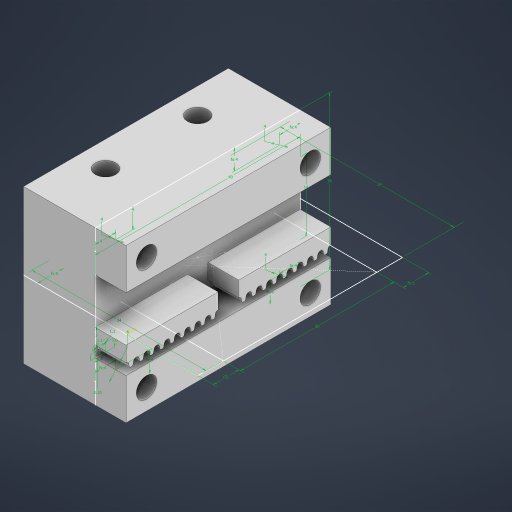
# Autodesk Inventor part: LRT_Back
Saved by Autodesk Inventor 2024.2 (Build 282272000, 272)
## iProperties
Created: 2024-09-29
Part Number: LRT_Back
Material: Generic
Document SubType Name: Modeling
Designer: jerem
Density: 1 g/cm^3
Appearance: Default
Author: jerem
## iProperties of the stored document linearRailToolhead_3DPrint.ipt
Created: 2024-09-29
Part Number: linearRailToolhead_3DPrint
Material: Generic
Document SubType Name: Modeling
Designer: jerem
Density: 1 g/cm^3
Appearance: Default
Author: jerem
Autodesk Inventor part; units mm, degrees
ref_plane "YZ Plane" through (0, 0, 0) normal (1, 0, 0) x (0, 1, 0)
ref_plane "XZ Plane" through (0, 0, 0) normal (0, 1, 0) x (-1, 0, 0)
ref_plane "XY Plane" through (0, 0, 0) normal (0, 0, 1) x (1, 0, 0)
sketch "Sketch1" plane through (0, 0, 0) normal (1, 0, 0) x (0, 1, 0)
  line L0 (-7, -20) -> (7, -20)
  line L1 (7, -20) -> (7, 20)
  line L2 (7, 20) -> (-7, 20)
  line L3 (-7, 20) -> (-7, -20)
  line L4 (7, -20) -> (1.25, -20)
  arc A0 (-5.3073, 19.4579) -> (-4.85, 20) centre (-5.4, 20) ccw
  arc A1 (-4.85, 18) -> (-5.3073, 18.5421) centre (-5.4, 18) ccw
  line L5 (-5.4, 20) -> (-5.4, 18) construction
  line L6 (-6, 19.1286) -> (-6, 18.8714)
  line L7 (-5.7921, 19.375) -> (-5.3073, 19.4579)
  line L8 (-5.3073, 18.5421) -> (-5.7921, 18.625)
  arc A2 (-5.7921, 19.375) -> (-6, 19.1286) centre (-5.75, 19.1286) ccw
  arc A3 (-6, 18.8714) -> (-5.7921, 18.625) centre (-5.75, 18.8714) ccw
  line L9 (-5.4, 18) -> (-4.85, 18) construction
  line L10 (-6, 19) -> (-5.4, 19) construction
  line L11 (-4.85, 18) -> (-1.85, 18)
  line L12 (-1.85, 18) -> (-1.85, 20)
  line L13 (7, -20) -> (-7, 20) construction
  line L14 (7, 20) -> (-7, -20) construction
  line L15 (7, 20) -> (15, 20)
  line L16 (15, 20) -> (15, -20)
  line L17 (15, -20) -> (7, -20)
  line L18 (-7, 20) -> (-15, 20)
  line L19 (-15, 20) -> (-15, -20)
  line L20 (-15, -20) -> (-7, -20)
  circle A4 centre (11, 16) radius 2
  circle A5 centre (11, -16) radius 2
  circle A6 centre (-11, 16) radius 2
  circle A7 centre (-11, -16) radius 2
  point P0 (0, 0)
  point P1 (0, 0)
  point P2 (11, 20)
  point P3 (-11, 20)
  dimension "d2" = 14
  dimension "d4" = 1.1
  dimension "d5" = 1.6
  dimension "d6" = 1.1
  dimension "d7" = 2
  dimension "d11" = 1
  dimension "d12" = 0.25
  dimension "d13" = 0.75
  dimension "d14" = 3
  dimension "d31" = 40
  dimension "d39" = 30
  dimension "d54" = 4
  dimension "d55" = 4
  dimension "d56" = 4
  dimension "d57" = 4
  dimension "d58" = 4
  dimension "d59" = 4
  dimension "d60" = 4
  dimension "d61" = 4
  dimension "d62" = 4
  dimension "d63" = 4
  dimension "d64" = 4
  dimension "d65" = 4
  constraints: 42 end point, 8 centre point, 8 point on circle, 6 perpendicular, 6 point on line, 6 tangent, 5 horizontal, 5 midpoint, 2 coincident, 2 parallel, 2 vertical, 1 collinear, 1 equal radius
  measures "d2" distance between parallel lines of L3 L1
  measures "d4" diameter of A0
  measures "d5" distance of L2.end L5.start
  measures "d6" diameter of A1
  measures "d7" distance of L5.end L5.start
  measures "d11" distance between parallel lines of L3 L6
  measures "d12" radius of A2
  measures "d13" distance of L8.end L7.start
  measures "d14" distance of L9.end L11.end
  measures "d31" distance of L0.end L1.end
  measures "d39" distance between parallel lines of L19 L16
  measures "d54" diameter of A4
  measures "d55" diameter of A5
  measures "d56" distance from line of L16 A4.centre
  measures "d57" distance of point (11, 20) A4.centre
  measures "d58" distance from line of L17 A5.centre
  measures "d59" diameter of A6
  measures "d60" diameter of A7
  measures "d61" distance from line of L20 A7.centre
  measures "d62" distance from line of L19 A7.centre
  measures "d63" distance from line of L19 A6.centre
  measures "d64" distance of point (-11, 20) A6.centre
  measures "d65" distance from line of L16 A5.centre
extrude "Extrusion1" add sketch "Sketch1" against normal blind 2 contours L3 L2 A0 L7 A2 L6 A3 L8 A1 L11 L12 L1 L0 | L2 L12 L11 A1 L8 A3 L6 A2 L7 A0
extrude "Extrusion2" add sketch "Sketch1" along normal blind 6 contours L2 L12 L11 A1 L8 A3 L6 A2 L7 A0
sketch "Sketch3" plane through (0, 0, 0) normal (0, 1, 0) x (-1, 0, 0)
  line L0 (0, 0) -> (-3, 0) construction
  line L1 (14, -15) -> (-20, -15)
  line L2 (-20, -15) -> (-20, 15)
  line L3 (-20, 15) -> (14, 15)
  line L4 (14, 15) -> (14, -15)
  line L5 (14, -15) -> (-20, 15) construction
  line L6 (-20, -15) -> (14, 15) construction
  line L7 (-6, 18) -> (-6, 20) projected
  line L8 (0, 20) -> (-6, 20) projected
  line L9 (-3, 20) -> (-3, 0) construction
  line L10 (14, -15) -> (14, -20)
  line L11 (14, -20) -> (-20, -20)
  line L12 (-20, -20) -> (-20, -15)
  line L13 (14, 15) -> (14, 20)
  line L14 (14, 20) -> (-20, 20)
  line L15 (-20, 20) -> (-20, 15)
  dimension "d29" = 34
  dimension "d30" = 30
  dimension "d36" = 5
  dimension "d37" = 5
  dimension "d44" = 34
  dimension "d45" = 5
  constraints: 28 end point, 4 perpendicular, 3 midpoint, 3 vertical, 2 horizontal, 2 parallel
  measures "d29" distance of L2.end L3.end
  measures "d30" distance of L1.end L2.end
  measures "d36" distance between parallel lines of L1 L11
  measures "d37" distance between parallel lines of L3 L8
  measures "d44" distance of L10.end L11.end
  measures "d45" distance between parallel lines of L3 L14
pattern_linear "Rectangular Pattern2" count 9 spacing 2 along (0, 0, -1) of "Extrusion2"
mirror "Mirror2" about plane through (0, 0, 0) normal (0, 0, 1) of "Extrusion2", "Rectangular Pattern2"
extrude "Extrusion4" add sketch "Sketch1" against normal blind 14 contours L3 L2 A0 L7 A2 L6 A3 L8 A1 L11 L12 L1 L0 | L20 L19 L18 L3 | L1 L15 L16 L17 | L2 L12 L11 A1 L8 A3 L6 A2 L7 A0 | A4 | A5 | A6 | A7
extrude "Extrusion5" add sketch "Sketch1" along normal up to surface (6 mm away) contours L20 L19 L18 L3 | L1 L15 L16 L17 | A4 | A5 | A6 | A7
sketch "Sketch4" plane through (-14, 15, 20) normal (0, 1, 0) x (1, 0, 0)
  circle A0 centre (29, 29) radius 2
  circle A1 centre (29, 11) radius 2
  circle A2 centre (5, 29) radius 2
  circle A3 centre (5, 11) radius 2
  line L0 (14, 40) -> (20, 40) projected
  line L1 (34, 40) -> (0, 40)
  line L2 (0, 40) -> (0, 0)
  line L3 (0, 0) -> (34, 0)
  line L4 (34, 0) -> (34, 40)
  line L5 (34, 0) -> (0, 40) construction
  line L6 (0, 0) -> (0, 40) construction
  line L7 (0, 0) -> (34, 40) construction
  line L8 (29, 29) -> (5, 29) construction
  line L9 (5, 29) -> (5, 11) construction
  line L10 (5, 11) -> (29, 11) construction
  line L11 (29, 11) -> (29, 29) construction
  line L12 (29, 29) -> (5, 11) construction
  line L13 (29, 11) -> (5, 29) construction
  point P0 (14, 20)
  point P1 (17, 20)
  point P2 (17, 20)
  dimension "d46" = 18
  dimension "d47" = 24
  dimension "d48" = 4
  dimension "d49" = 4
  dimension "d50" = 4
  dimension "d51" = 4
  constraints: 24 end point, 4 centre point, 4 parallel, 3 coincident, 2 horizontal, 2 midpoint, 2 perpendicular, 2 other
  measures "d46" distance of A1.centre L8.start
  measures "d47" distance of L9.end L10.end
  measures "d48" diameter of A0
  measures "d49" diameter of A1
  measures "d50" diameter of A3
  measures "d51" diameter of A2
extrude "Extrusion6" cut sketch "Sketch4" against normal blind 3 contours A2 | A3
mirror "Mirror3" about plane through (0, 0, 0) normal (0, 1, 0) of "Extrusion6"
extrude "Extrusion7" cut sketch "Sketch1" against normal blind 6 from surface at 6 contours A4 | A5 | A6 | A7
equation "\"d58\" = d57"
equation "\"d61\" = d58"
equation "\"d62\" = d56"
equation "\"d63\" = d54"
equation "\"d64\" = d57"
equation "\"d65\" = d54"
equation "\"d36\" = d37"
equation "\"d45\" = d37"
equation "\"d49\" = d48"
equation "\"d50\" = d48"
equation "\"d51\" = d48"
body "Solid1"
